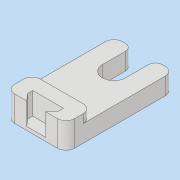
# Autodesk Inventor part: HallEffectSpoolSensorMount3
Saved by Autodesk Inventor 2017.3 (Build 213256000, 256)
## iProperties
Created: 2018-04-12
Part Number: HallEffectSpoolSensorMount3
Material: ABS Plastic
Document SubType Name: Modeling
Designer: Derek Wider
Density: 1.06 g/cm^3
Appearance: Smooth - White
Author: Derek Wider
Autodesk Inventor part; units mm, degrees
ref_plane "YZ Plane" through (0, 0, 0) normal (1, 0, 0) x (0, 1, 0)
ref_plane "XZ Plane" through (0, 0, 0) normal (0, 1, 0) x (-1, 0, 0)
ref_plane "XY Plane" through (0, 0, 0) normal (0, 0, 1) x (1, 0, 0)
sketch "Sketch1" plane through (0, 0, 0) normal (0, 1, 0) x (-1, 0, 0)
  line L0 (0, 0) -> (8.89, 0)
  line L1 (8.89, 0) -> (8.89, -16.002)
  line L2 (8.89, -16.002) -> (0, -16.002)
  line L3 (0, -16.002) -> (0, 0)
  dimension "d0" = 8.89
  dimension "d1" = 16.002
  constraints: 8 end point, 2 parallel, 1 horizontal, 1 perpendicular
  measures "d0" distance of L0.start L0.end
  measures "d1" distance of L0.end L1.end
extrude "Extrusion1" add sketch "Sketch1" along normal blind 2.54
sketch "Sketch5" plane through (0, 2.54, 0) normal (0, 1, 0) x (1, 0, 0)
  line L0 (-8.89, 0) -> (0, 0) projected
  line L1 (0, 0) -> (0, 16.002) projected
  line L2 (0, 16.002) -> (-8.89, 16.002) projected
  line L3 (-8.89, 16.002) -> (-8.89, 0) projected
  line L4 (0, 0) -> (-8.89, 0) projected
  line L5 (-5.842, 0) -> (-6.731, 1.016)
  line L6 (-6.731, 1.016) -> (-6.731, 1.778)
  line L7 (-6.731, 1.778) -> (-2.159, 1.778)
  line L8 (-2.159, 1.778) -> (-2.159, 1.016)
  line L9 (-2.159, 1.016) -> (-3.048, 0)
  line L10 (-8.89, 0) -> (-8.89, 16.002) projected
  line L11 (-8.89, 3.81) -> (0, 3.81)
  point P0 (-4.445, 1.778)
  point P1 (-4.445, 3.81)
  dimension "d19" = 2.794
  dimension "d20" = 4.572
  dimension "d21" = 1.016
  dimension "d23" = 1.778
  dimension "d24" = 3.81
  constraints: 12 end point, 4 perpendicular, 4 point on line, 2 midpoint, 1 equal length, 1 horizontal alignment, 1 vertical alignment
  measures "d19" distance of L9.end L5.start
  measures "d20" distance of L6.end L7.end
  measures "d21" vertical distance of L9.end L8.end
  measures "d23" distance between parallel lines of L0 L7
  measures "d24" distance between parallel lines of L0 L11
extrude "Extrusion4" add sketch "Sketch5" along normal blind 1.27 contours L3 L11 L1 L0 L9 L8 L7 L6 L5
sketch "Sketch6" plane through (0, 2.54, 0) normal (0, 1, 0) x (1, 0, 0)
  line L0 (-3.048, 0) -> (-2.159, 1.016) projected
  line L1 (-2.159, 1.016) -> (-2.159, 1.778) projected
  line L2 (-2.159, 1.778) -> (-6.731, 1.778) projected
  line L3 (-6.731, 1.778) -> (-6.731, 1.016) projected
  line L4 (-6.731, 1.016) -> (-5.842, 0) projected
  line L5 (-5.842, 0) -> (-3.048, 0) projected
  point P0 (0, 0)
extrude "Extrusion5" cut sketch "Sketch6" against normal blind 2.032
fillet "Fillet3" radius 1.27 6 edges at (-8.89, 1.27, -16.002) (0, 1.27, -16.002) (-8.89, 1.905, 0) (-8.89, 3.175, -3.81) (0, 3.175, -3.81) (0, 1.905, 0)
sketch "Sketch8" plane through (0, 2.54, 0) normal (0, 1, 0) x (1, 0, 0)
  line L0 (-7.62, 16.002) -> (-1.27, 16.002) projected
  line L1 (-6.1595, 16.002) -> (-6.1595, 11.557)
  line L2 (-2.7305, 16.002) -> (-2.7305, 11.557)
  arc A0 (-6.1595, 11.557) -> (-2.7305, 11.557) centre (-4.445, 11.557) ccw
  point P0 (0, 0)
  point P1 (-4.445, 16.002)
  dimension "d37" = 3.429
  dimension "d38" = 4.445
  constraints: 4 end point, 2 point on circle, 2 point on line, 2 tangent, 1 centre point, 1 midpoint, 1 perpendicular, 1 vertical, 1 vertical alignment
  measures "d37" distance between parallel lines of L2 L1
  measures "d38" distance from line of L0 A0.centre
extrude "Extrusion7" cut sketch "Sketch8" against normal blind 25.4
fillet "Fillet4" radius 1.016 2 edges at (-2.7305, 1.27, -16.002) (-6.1595, 1.27, -16.002)
body "Solid1"
